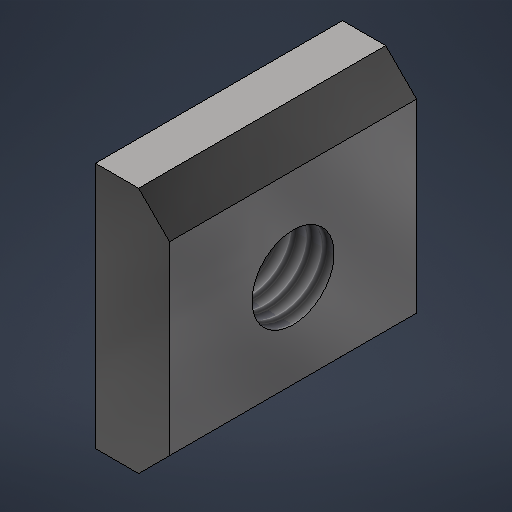
# Autodesk Inventor part: NUT, MK 1, M8
Saved by Autodesk Inventor 2026.1 (Build 301233020, 233B)
## iProperties
Manager: 100-30419
Category: _
Material: Steel, Alloy
Document SubType Name: Modeling
Created: 2023-04-20
Designer: keithl , Keith
Manufacturer: Standard
Standards Organization: Custom
Checked By: 1DN68
User Status: Work In Process
Description: NUT, MK 1, M8
Engr Approved By: R
Mass: 15.9763 g
Surface Area: 12.6481 cm^2
Volume: 2.06679 cm^3
Density: 7.73 g/cm^3
Mfg Approved By: Cathy.Lesperance
Appearance: Semi-Polished
Part Number: NUT, MK 1, M8
Control State: 0
Master: False
Checked Out: False
Shininess: 64.0
Angle Display Precision: 2
Document Length Units: 11269
Document Angle Units: 11279
Document Time Units: 11290
Document Mass Units: 11286
Document Length Units Precision: 3
Document Angle Units Precision: 2
Translation Standard: STEP AP214DIS
File Name: //partserver001.servicenet/client_exchange/iodir/jobs/output/wkb8294379_no0/STEP/34_01_0001_2_14a.stp
Postprocessor: Build: 081d, Release: 8 SP1 - Date: Tue 01/26/2004
Sent Units: MILLIMETERS
Uncertainty: 1.0000000000000002e-06
CN_SERVICEABLE: _
FIRST_DESCRIPTION: NUT, MK 1, M8
PTC_WM_ITERATION: 9
PTC_WM_ORGANIZATION_ID: CLWC
PTC_WM_LIFECYCLE: CLWC_CAD_LC
CN_MASS: 0.02
CL_runCount: 1
FinishProperty: ToBeSet
SECOND_DESCRIPTION: _
THIRD_DESCRIPTION: _
CUSTOMERNUMBER: _
ModelCat: Uncategorized
Density: 0.0
Volumn: 0.0
Area: 0.0
PropertySet Name: Model Information
Subject: 34.01.0001
Keywords: MK
Revision Number: 1
Author: -
Autodesk Inventor part; units mm, degrees
ref_plane "YZ Plane" through (0, 0, 0) normal (1, 0, 0) x (0, 1, 0)
ref_plane "XZ Plane" through (0, 0, 0) normal (0, 1, 0) x (-1, 0, 0)
ref_plane "XY Plane" through (0, 0, 0) normal (0, 0, 1) x (1, 0, 0)
sketch "Sketch2" plane through (0, 0, 0) normal (0, 0, 1) x (1, 0, 0)
  line L0 (0, -10) -> (3.5, -10)
  line L1 (0, 10) -> (0, -10)
  line L2 (3.5, 10) -> (0, 10)
  line L3 (6, 7.5) -> (3.5, 10)
  line L4 (6, -7.5) -> (6, 7.5)
  line L5 (3.5, -10) -> (6, -7.5)
  line L6 (-1.2, 0) -> (7.2, 0) construction
  line L7 (0, -14) -> (0, 14) construction
  dimension "d11" = 20
  dimension "d12" = 15
  dimension "d13" = 45
  dimension "d14" = 6
  constraints: 12 end point, 1 collinear, 1 perpendicular, 2 other
  measures "d11" distance of L1.start L0.start
  measures "d12" distance of L4.start L3.start
  measures "d13" angle of L0 L5
  measures "d14" distance between parallel lines of L1 L4
extrude "Extrusion2" add sketch "Sketch2" along normal mid plane 20
hole "Hole1" at (0, 0, 0) direction (1, 0, 0) diameter 6.647 end through all thread size "M8x1.25" class "6H" standard "ANSI Metric M Profile"
body "Solid2"
